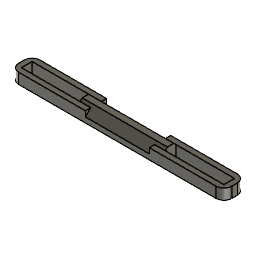
camera holder (Autodesk Fusion 360 design; units mm, degrees)
part number: 2026-02-28-01-15-09-460
Autodesk Fusion 360 part; units mm, degrees
sketch "Sketch1" plane through (0, 0, 0) normal (0, 0, 1) x (1, 0, 0)
  line L0 (0, 0) -> (200, 0)
  line L1 (200, 0) -> (200, 20)
  line L2 (200, 20) -> (0, 20)
  line L3 (0, 20) -> (0, 0)
  line L4 (100, 20) -> (130, 20)
  line L5 (130, 20) -> (130, 0)
  line L6 (130, 0) -> (100, 0)
  line L7 (100, 0) -> (100, 20)
  line L8 (130, 0) -> (70, 0)
  line L9 (70, 0) -> (70, 20)
  line L10 (70, 20) -> (130, 20)
  line L11 (130, 20) -> (130, 0)
  line L12 (140, 15) -> (195, 15)
  line L13 (195, 15) -> (195, 5)
  line L14 (195, 5) -> (140, 5)
  line L15 (140, 5) -> (140, 15)
  line L16 (60, 5) -> (5, 5)
  line L17 (5, 5) -> (5, 15)
  line L18 (5, 15) -> (60, 15)
  line L19 (60, 15) -> (60, 5)
  dimension "d1" = 200
  dimension "d2" = 20
  constraint horizontal L0
  constraint vertical L1
  constraint horizontal L2
  constraint vertical L3
  constraint coincident L0.start L3.end
  constraint horizontal L4
  constraint vertical L5
  constraint horizontal L6
  constraint vertical L7
  constraint coincident L0 L5.end
  constraint midpoint L2 L4.start
  constraint horizontal L8
  constraint vertical L9
  constraint horizontal L10
  constraint vertical L11
  constraint coincident L2 L9.end
  constraint horizontal L12
  constraint vertical L13
  constraint horizontal L14
  constraint vertical L15
  constraint horizontal L16
  constraint vertical L17
  constraint horizontal L18
  constraint vertical L19
  measures "d1" distance of L0.start L0.end
  measures "d2" distance of L0.start L2.end
extrude "Extrude1" add sketch "Sketch1" along normal blind 10
fillet "Fillet1" radius 7.5 4 edges at (200, 20, 5) (200, 0, 5) (0, 0, 5) (0, 20, 5)
sketch "Sketch2" plane through (0, 0, 10) normal (0, 0, 1) x (-1, 0, 0)
  arc A0 (-7.5, -20) -> (0, -12.5) centre (-7.5, -12.5) ccw
  line L0 (0, -12.5) -> (0, -7.5)
  arc A1 (0, -7.5) -> (-7.5, 0) centre (-7.5, -7.5) ccw
  line L1 (-7.5, 0) -> (-192.5, 0)
  arc A2 (-192.5, 0) -> (-200, -7.5) centre (-192.5, -7.5) ccw
  line L2 (-200, -7.5) -> (-200, -12.5)
  arc A3 (-200, -12.5) -> (-192.5, -20) centre (-192.5, -12.5) ccw
  line L3 (-192.5, -20) -> (-7.5, -20)
  line L4 (-195, -5) -> (-140, -5)
  line L5 (-140, -5) -> (-140, -15)
  line L6 (-140, -15) -> (-195, -15)
  line L7 (-195, -15) -> (-195, -5)
  line L8 (-5, -15) -> (-60, -15)
  line L9 (-60, -15) -> (-60, -5)
  line L10 (-60, -5) -> (-5, -5)
  line L11 (-5, -5) -> (-5, -15)
  line L12 (-60, -20) -> (-140, -20)
  line L13 (-140, -20) -> (-140, 0)
  line L14 (-140, 0) -> (-60, 0)
  line L15 (-60, 0) -> (-60, -20)
  constraint horizontal L12
  constraint vertical L13
  constraint horizontal L14
  constraint vertical L15
  constraint coincident L1 L13.end
  constraint coincident L3 L12.start
extrude "Extrude2" add sketch "Sketch2" along normal blind 2 contours L1 L3 L5 L9 L12 L13 L14 L15
extrude "Extrude3" cut 2 faces at (24.1667, 3.3333, 10) (175.8333, 3.3333, 10) along direction (0, 0, -1) blind 10
chamfer "Chamfer1" distance 7 angle 45 2 edges at (100, 0, 12) (100, 20, 12)
extrude "Extrude4" add sketch "Sketch1" along normal blind 10 contours L0 L2 L3 L9 | L0 L1 L2 L5 L11
fillet "Fillet2" radius 7.5 4 edges at (0, 20, 5) (0, 0, 5) (200, 20, 5) (200, 0, 5)
